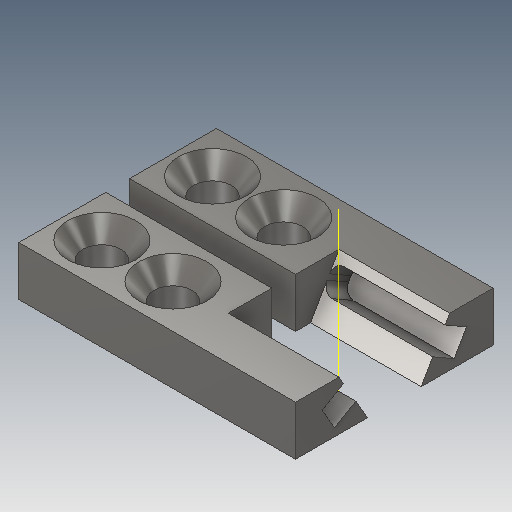
# Autodesk Inventor part: v2_bearing_insert_thick_parallel_REF
Saved by Autodesk Inventor 2019 (Build 230136000, 136)
## iProperties
Created: 2017-04-27
Part Number: v2_bearing_insert_thick_parallel_REF
Material: Stainless Steel, 440C
Document SubType Name: Modeling
Designer: richp
Density: 7.75 g/cm^3
Appearance: Semi-Polished
bearing_thickness: 0.125 in
bearing_angle: 60.00 deg
bearing_spacing: 0.068 in
flat_bearing_surface_height: 0.110 in
hole1_setback: 0.280 in
hole2_setback: 0.460 in
hole_lateral: 0.140 in
carbide_insert_width: 0.063 in
Author: richp
Autodesk Inventor part; units mm, degrees
ref_plane "YZ Plane" through (0, 0, 0) normal (1, 0, 0) x (0, 1, 0)
sketch "Sketch1" plane through (0, 0, 0) normal (1, 0, 0) x (0, 1, 0)
  line L0 (-2.2042, 0) -> (7.9897, 0) construction
  line L1 (0, -10.9768) -> (0, 10.9768) construction
  line L2 (0, -1.7272) -> (0, -6.35)
  line L3 (0, -1.7272) -> (0, -1.7272)
  line L4 (0, -1.7272) -> (3.175, -3.5603)
  line L5 (3.175, -3.5603) -> (3.175, -6.35)
  line L6 (3.175, -6.35) -> (0, -6.35)
  circle A0 centre (3.3584, 0) radius 3.175 construction
  line L7 (2.5647, 7.8406) -> (4.1522, 7.8406) construction
  line L8 (4.1522, 7.8406) -> (4.1522, -7.8406) construction
  line L9 (4.1522, -7.8406) -> (2.5647, -7.8406) construction
  line L10 (2.5647, -7.8406) -> (2.5647, 7.8406) construction
  line L11 (2.5647, 7.8406) -> (4.1522, -7.8406) construction
  line L12 (4.1522, 7.8406) -> (2.5647, -7.8406) construction
  line L13 (0, 1.7272) -> (0, 6.35)
  line L14 (0, 1.7272) -> (0, 1.7272)
  line L15 (0, 1.7272) -> (3.175, 3.5603)
  line L16 (3.175, 3.5603) -> (3.175, 6.35)
  line L17 (3.175, 6.35) -> (0, 6.35)
  point P0 (0, 0)
  point P1 (2.3851, -3.0222)
  point P2 (2.3851, 3.0222)
  point P3 (1.7709, 2.7496)
  point P4 (1.7709, -2.7496)
  dimension "bearing_angle" = 60
  dimension "d13" = 0
  dimension "bearing_thickness" = 3.175
  dimension "bearing_spacing" = 1.7272
  dimension "d17" = 6.35
  dimension "d18" = 1.5875
  dimension "d23" = 12.7
  dimension "d52" = 3.3584
  dimension "d78" = 0.3668
  dimension "flat_bearing_surface_height" = 2.794
  constraints: 32 end point, 5 symmetric about line, 4 perpendicular, 4 point on circle, 4 point on line, 2 horizontal, 2 midpoint, 2 parallel, 1 centre point, 1 coincident, 1 tangent
  measures "bearing_angle" angle of L1 L4
  measures "d13" distance of L2.start L3.end
  measures "bearing_thickness" distance of L5.end L2.end
  measures "bearing_spacing" distance from line of point (0, 0) L3
  measures "d17" diameter of A0
  measures "d18" distance between parallel lines of L10 L8
  measures "d23" distance between parallel lines of L6 L17
  measures "d52" distance from line of L2 A0.centre
sketch "Sketch11" plane through (0, 0, 0) normal (1, 0, 0) x (0, 1, 0)
  line L0 (3.175, 6.35) -> (0, 6.35) projected
  line L1 (3.175, -6.35) -> (0, -6.35) projected
  line L2 (-2.2042, 0) -> (7.9897, 0) construction
  line L3 (0, -10.9768) -> (0, 10.9768) construction
  line L4 (3.175, 6.35) -> (3.175, 0.762)
  line L5 (3.175, 0.762) -> (0, 0.762)
  line L6 (0, 6.35) -> (0, 0.762)
  line L7 (3.175, -6.35) -> (0, -6.35)
  line L8 (0, 10.9768) -> (0, -10.9768) construction
  line L9 (3.175, -6.35) -> (3.175, -0.762)
  line L10 (3.175, -0.762) -> (0, -0.762)
  line L11 (0, -6.35) -> (0, -0.762)
  point P0 (0, 0)
  dimension "d54" = 5.588
  constraints: 16 end point, 4 symmetric about line, 2 perpendicular, 2 point on line, 1 vertical
  measures "d54" distance of L0.start L4.end
extrude "Extrusion4" add sketch "Sketch11" along normal blind 3.556 and the other way blind 14.224
sketch "Sketch17" plane through (3.556, 0, 0) normal (1, 0, 0) x (0, 0, -1)
  line L0 (-6.35, 3.175) -> (-0.762, 3.175) projected
  line L1 (-0.762, 3.175) -> (0.762, 3.175)
  line L2 (0.762, 3.175) -> (0.762, 0)
  line L3 (0.762, 0) -> (-0.762, 0)
  line L4 (-0.762, 0) -> (-0.762, 3.175)
  point P0 (0, 0)
  constraints: 8 end point, 2 parallel, 1 horizontal, 1 perpendicular
ref_plane "Work Plane3" through (0, 3.175, 6.35) normal (1, 0, 0) x (0, -1, 0)
extrude "Extrusion6" [suppressed]
sketch "Sketch14" plane through (-14.224, 3.175, -6.35) normal (0, 1, 0) x (1, 0, 0)
  line L0 (-3.556, -6.35) -> (21.336, -6.35) projected
  line L1 (0, -5.588) -> (0, 0) projected
  point P0 (14.224, -6.35)
  point P1 (2.54, -2.794)
  point P2 (7.112, -2.794)
  point P3 (2.54, -9.906)
  point P4 (7.112, -9.906)
  dimension "hole1_setback" = 7.112
  dimension "hole2_setback" = 11.684
  dimension "hole_lateral" = 3.556
  constraints: 2 symmetric about line, 1 horizontal alignment
  measures "hole1_setback" horizontal distance of point (7.112, -2.794) point (14.224, -6.35)
  measures "hole2_setback" horizontal distance of point (2.54, -2.794) point (14.224, -6.35)
  measures "hole_lateral" distance from line of L0 point (2.54, -2.794)
hole "Hole2" at (-11.684, 3.175, -3.556) at (-7.112, 3.175, -3.556) at (-11.684, 3.175, 3.556) at (-7.112, 3.175, 3.556) direction (0, -1, 0) diameter 2.4384 depth 6.6294 tip angle 118 countersink diameter 4.3688 countersink angle 82 clearance for "Flat Head Machine Screw (82)" size "#2" standard "Ansi Unified Screw Threads"
sketch "Sketch12" plane through (0, 3.175, 6.35) normal (1, 0, 0) x (0, -1, 0)
  line L0 (3.175, 4.6228) -> (0, 2.7897) projected
  line L1 (3.175, 8.0772) -> (0, 9.9103) projected
  line L2 (5.3792, 6.35) -> (-4.8147, 6.35) construction
  line L3 (3.175, 17.3268) -> (3.175, -4.6268) construction
  line L4 (3.175, 4.6228) -> (3.175, 7.0113)
  line L5 (3.175, 4.6228) -> (3.175, 4.6228)
  line L6 (3.175, 8.0772) -> (3.175, 8.0772)
  line L7 (3.175, 7.0113) -> (3.175, 8.0772)
  line L8 (0, 2.7897) -> (0, 9.9103)
  line L9 (0, 0) -> (0, 5.588) projected
  point P0 (3.175, 6.35)
  constraints: 10 end point, 4 collinear, 3 point on line
extrude "Extrusion5" cut sketch "Sketch12" along normal mid plane 7.112
ref_plane "Work Plane4" through (0, 2.5647, -7.8406) normal (-1, 0, 0) x (0, 0, 1)
revolve "Revolution7" [suppressed]
sketch "Sketch13" plane through (0, 3.175, 6.35) normal (1, 0, 0) x (0, -1, 0)
  circle A0 centre (-0.1834, 6.35) radius 3.175 projected
  line L0 (5.3792, 6.35) -> (-4.8147, 6.35) construction
  line L1 (-3.3584, 6.35) -> (2.9916, 6.35)
  point P0 (3.175, 6.35)
  constraints: 2 end point, 2 point on circle, 2 point on line
revolve "Revolution6" [suppressed]
sketch "Sketch18" plane through (-3.556, 3.175, -3.5603) normal (0, 0.5, 0.866) x (1, 0, 0)
  circle A0 centre (3.556, -1.6213) radius 1.5748
  point P0 (3.556, -4.5298)
  point P1 (3.556, -1.6213)
  dimension "d80" = 3.1496
  constraints: 1 centre point, 1 coincident
  measures "d80" diameter of A0
sketch "Sketch19" plane through (3.556, 0, 0) normal (1, 0, 0) x (0, 0, -1)
  circle A0 centre (3.437, 1.374) radius 0.7937
  line L0 (3.5603, 3.175) -> (1.7272, 0) projected
  point P0 (0, 0)
  point P1 (2.7496, 1.7709)
  dimension "d81" = 1.5875
  constraints: 4 other
sketch "Sketch20" plane through (-3.556, 3.175, -3.5603) normal (0, 0.5, 0.866) x (1, 0, 0)
  line L0 (0, 0.1438) -> (0, -3.6662) projected
  line L1 (7.112, 0) -> (7.112, -3.6662) projected
  line L2 (0, 0.1438) -> (7.112, 0.1438)
  line L3 (7.112, 0.1438) -> (7.112, -3.6662)
  line L4 (7.112, -3.6662) -> (0, -3.6662)
  line L5 (0, -3.6662) -> (0, 0.1438)
  point P0 (3.556, -4.5298)
  dimension "d86" = 3.81
  constraints: 9 end point, 2 parallel, 1 horizontal, 1 perpendicular
  measures "d86" distance between parallel lines of L2 L4
extrude "Extrusion7" [suppressed]
extrude "Extrusion8" [suppressed]
sketch "Sketch21" plane through (3.556, 0, 0) normal (1, 0, 0) x (0, 0, -1)
  line L0 (-1.7272, 0) -> (-3.5603, 3.175) projected
  line L1 (-3.267, 2.667) -> (-2.4732, 1.2922)
  line L2 (-2.4732, 1.2922) -> (-3.8481, 0.4984)
  line L3 (-3.8481, 0.4984) -> (-4.6418, 1.8732)
  line L4 (-4.6418, 1.8732) -> (-3.267, 2.667)
  line L5 (0, -2.2042) -> (0, 7.9897) projected
  line L6 (3.267, 2.667) -> (2.4732, 1.2922)
  line L7 (2.4732, 1.2922) -> (3.8481, 0.4984)
  line L8 (3.8481, 0.4984) -> (4.6418, 1.8732)
  line L9 (4.6418, 1.8732) -> (3.267, 2.667)
  point P0 (0, 0)
  dimension "carbide_insert_width" = 1.5875
  dimension "d88" = 1.5875
  dimension "d89" = 0.508
  constraints: 16 end point, 4 symmetric about line, 2 parallel, 2 point on line, 1 perpendicular
  measures "carbide_insert_width" distance between parallel lines of L2 L4
  measures "d88" distance between parallel lines of L3 L1
  measures "d89" vertical distance of L0.end L1.start
extrude "Extrusion9" cut sketch "Sketch21" against normal blind 7.112
fillet "Fillet1" radius 0.635 4 edges at (-3.556, 2.2701, -3.9544) (-3.556, 0.8953, -3.1607) (-3.556, 0.8953, 3.1607) (-3.556, 2.2701, 3.9544)
sketch "Sketch16" plane through (0, 2.5647, -7.8406) normal (-1, 0, 0) x (0, 0, 1)
  line L0 (6.1134, -2.5647) -> (4.2803, 0.6103) projected
  line L1 (9.5678, -2.5647) -> (11.4008, 0.6103) projected
  line L2 (11.4008, 0.6103) -> (4.2803, 0.6103) projected
  line L3 (7.1793, -2.5647) -> (6.1134, -2.5647) projected
  line L4 (9.5678, -2.5647) -> (7.1793, -2.5647) projected
  line L5 (9.5678, -2.5647) -> (9.5678, -2.5647)
  line L6 (6.1134, -2.5647) -> (6.1134, -2.5647)
  line L7 (7.8406, -4.7688) -> (7.8406, 5.425) projected
  line L8 (7.8406, 0.6103) -> (7.8406, -2.5647)
  constraints: 6 end point, 1 collinear, 1 midpoint, 1 point on line
body "Solid2"
